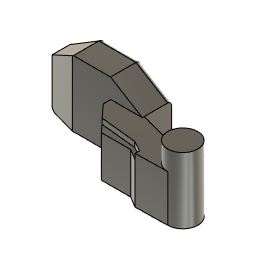
primary_015mm_trigger_L1 (Autodesk Fusion 360 design; units mm, degrees)
Autodesk Fusion 360 part; units mm, degrees
other "Base Mesh Feature1"
sketch "Sketch1" plane through (0, 0, 0) normal (0, 0, 1) x (1, 0, 0)
  circle A0 centre (0, 0) radius 1
  dimension "d1" = 2
  constraint coincident A0.centre origin
  measures "d1" diameter of A0
other "Modify1"
ref_plane "WorkPlane1" through (0, 6, 0) normal (0, 1, 0) x (0, 0, 1)
sketch "Sketch2" plane through (0, 6, 0) normal (0, 1, 0) x (1, 0, 0)
  line L0 (1.6523, 0) -> (-15.6516, 0)
  line L1 (-16.1535, -0.5035) -> (-16.1535, -9.0095)
  line L2 (-10.7208, -12.3222) -> (-3.7767, -12.3222)
  line L3 (2.15, -8.7069) -> (2.15, -0.4961)
  line L4 (2.15, -8.7069) -> (-3.7767, -12.3222)
  line L5 (-10.7208, -12.3222) -> (-16.1535, -9.0095)
  line L6 (-16.1535, -0.5035) -> (-15.6516, 0)
  line L7 (1.6523, 0) -> (2.15, -0.4961)
  constraint horizontal L0
  constraint vertical L1
  constraint horizontal L2
  constraint vertical L3
  constraint perpendicular L6 L7
extrude "Extrude1" add sketch "Sketch2" against normal blind 6 makes body 1
sketch "Sketch3" plane through (0, 0, 0) normal (0, 0, 1) x (1, 0, 0)
  line L0 (3.6212, 0.4483) -> (3.7132, 0.4483)
  line L1 (-3.7364, -0.8889) -> (-3.7364, 0.4483)
  line L2 (7.233, -5.95) -> (5.2372, -4.7374)
  line L3 (-0.2601, -4.7374) -> (5.2372, -4.7374)
  line L4 (-3.7364, -0.8889) -> (-0.2601, -4.7374)
  line L5 (3.6212, 0.4483) -> (3.6212, 0.473)
  line L6 (0.7678, 1.2417) -> (-3.7364, 1.2417)
  line L7 (-3.7364, 1.2417) -> (-3.7364, 0.4483)
  circle A0 centre (13.2416, -3.0159) radius 2.8307
  line L8 (10.8649, -1.4783) -> (0.4006, 1.3406)
  line L9 (7.233, -5.95) -> (13.2901, -5.8462)
  constraint horizontal L0
  constraint vertical L1
  constraint horizontal L3
  constraint vertical L5
  constraint horizontal L6
  constraint vertical L7
  constraint coincident A0 L8.start
  constraint coincident L8 L0.end
  constraint coincident L8 L5.end
  constraint coincident L8 L6.start
  constraint coincident A0 L9.end
  constraint tangent A0 L9
extrude "Extrude2" add sketch "Sketch3" along normal blind 8.7 separate body contours L0 L1 L2 L3 L4 L5 L6 L7 A0 L8 L9 makes body 2
extrude "Extrude3" add sketch "Sketch3" along normal blind 12.35 separate body contours A0 makes body 3
sketch "Sketch4" plane through (0, 0, 0) normal (0, 0, 1) x (1, 0, 0)
ref_plane "WorkPlane2" through (0, 0, 8.7) normal (0, 0, 1) x (1, 0, 0)
sketch "Sketch5" plane through (0, 0, 8.7) normal (0, 0, 1) x (1, 0, 0)
  line L0 (-1.6701, -3.3156) -> (5.2766, -4.0362)
  line L1 (5.2766, -4.0362) -> (7.2469, -5.1058)
  line L2 (7.2469, -5.1058) -> (7.2469, -8)
  line L3 (7.2469, -8) -> (-2, -8)
  line L4 (-2, -8) -> (-2, -3.2819)
  line L5 (-2, -3.2819) -> (-1.6701, -3.3156)
  constraint vertical L2
  constraint perpendicular L2 L3
  constraint perpendicular L3 L4
extrude "Extrude4" cut sketch "Sketch5" against normal blind 1 bodies 2
fillet "Fillet1" radius 0.75 3 edges at (-0.8134, 6, 10.5146) (-7.2488, 6, 12.3222) (-13.4372, 6, 10.6658) on bodies 1
extrude "Extrude5" cut 1 faces at (-5.9253, 0, 4.1074) along direction (0, 1, 0) blind 0.5 on bodies 1 bodies 1 2
sketch "Sketch6" plane through (0, 0, 0) normal (0, 0, 1) x (1, 0, 0)
  line L0 (-10.6703, 0.4352) -> (-16.4272, 2.0156)
  line L1 (-16.4272, 2.0156) -> (-16.4272, 0.4352)
  line L2 (-16.4272, 0.4352) -> (-10.6703, 0.4352)
  constraint vertical L1
  constraint perpendicular L1 L2
extrude "Extrude6" cut sketch "Sketch6" along normal blind 15 bodies 1
sketch "Sketch7" plane through (0, 0, 8.7) normal (0, 0, 1) x (-1, 0, 0)
  line L0 (-2.15, 0) -> (3.7364, 0)
  line L1 (3.7364, 0) -> (3.7364, 0.8889)
  line L2 (3.7364, 0.8889) -> (1.5314, 3.33)
  line L3 (1.5314, 3.33) -> (-5.2766, 4.0362)
  line L4 (-5.2766, 4.0362) -> (-7.2469, 5.1058)
  line L5 (-7.2469, 5.1058) -> (-7.2469, 5.9498)
  line L6 (-7.2469, 5.9498) -> (-13.2901, 5.8462)
  arc A0 (-10.8649, 1.4783) -> (-13.2901, 5.8462) centre (-13.2416, 3.0159) ccw
  line L7 (-10.8649, 1.4783) -> (-3.7132, -0.4483)
  line L8 (-3.7132, -0.4483) -> (-3.6212, -0.4483)
  line L9 (-3.6212, -0.4483) -> (-3.6212, -0.473)
  line L10 (-3.6212, -0.473) -> (-0.7678, -1.2417)
  line L11 (-0.7678, -1.2417) -> (3.7364, -1.2417)
  line L12 (3.7364, -1.2417) -> (3.7364, -0.5)
  line L13 (3.7364, -0.5) -> (-2.15, -0.5)
  line L14 (-2.15, -0.5) -> (-2.15, 0)
  line L15 (-2.15, 0) -> (3.7364, 0)
  line L16 (3.7364, 0) -> (3.7364, -0.5)
  line L17 (3.7364, -0.5) -> (-2.15, -0.5)
  line L18 (-2.15, -0.5) -> (-2.15, 0)
  constraint horizontal L15
  constraint vertical L16
  constraint horizontal L17
  constraint vertical L18
  constraint coincident L12.end L13.start
  constraint coincident L0.start L14.end
extrude "Extrude7" add sketch "Sketch7" against normal blind 8.7 contours L0 L13 L14 L15 L16 L17 L18 bodies 2 1
combine "Combine1" operation add target body 2 tool bodies 3
